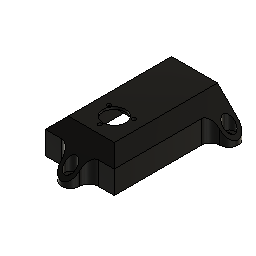
V205 Drybox Connector Buddy v2 (Autodesk Fusion 360 design; units mm, degrees)
Autodesk Fusion 360 part; units mm, degrees
sketch "Sketch7" plane through (0, 0, 0) normal (0, 0, 1) x (1, 0, 0)
  line L0 (30, -50) -> (-30, -50)
  line L1 (-30, -50) -> (-30, 50)
  line L2 (-30, 50) -> (30, 50)
  line L3 (30, 50) -> (30, -50)
  line L4 (30, -50) -> (-30, 50) construction
  line L5 (-30, -50) -> (30, 50) construction
  dimension "d21" = 60
  dimension "d22" = 100
  constraint horizontal L0
  constraint perpendicular L0 L1
  constraint parallel L0 L2
  constraint parallel L1 L3
  constraint coincident L4 origin
  constraint coincident L5 origin
  measures "d21" distance of L1.end L2.end
  measures "d22" distance of L0.end L1.end
extrude "Extrude13" add sketch "Sketch7" along normal blind 30 makes body 1
chamfer "Chamfer8" distance 10 angle 45 3 edges at (-30, 0, 30) (30, 0, 30) (0, -50, 30) tangent chain off on bodies 1
shell "Shell2" thickness 2 removed faces 1 at (-10, 16.6667, 0) on bodies 1
ref_plane "WorkPlane2" through (0, 0, 20) normal (0, 0, 1) x (1, 0, 0)
sketch "Sketch8" plane through (0, 0, 20) normal (0, 0, 1) x (1, 0, 0)
  line L0 (30, 50) -> (30, -50)
  line L1 (30, -50) -> (-30, -50)
  line L2 (-30, -50) -> (-30, 50)
  line L3 (-30, 50) -> (30, 50)
  line L4 (0, -50) -> (0, -58) construction
  circle A0 centre (0, -58) radius 8 construction
  circle A1 centre (38, 42) radius 8 construction
  circle A2 centre (-38, 42) radius 8 construction
  line L5 (30, 50) -> (38, 50)
  line L6 (-30, 50) -> (-38, 50)
  line L7 (38, 34) -> (30, 34)
  line L8 (-38, 34) -> (-30, 34)
  line L9 (8, -58) -> (8, -50)
  line L10 (-8, -58) -> (-8, -50)
  line L11 (8, -50) -> (-8, -50)
  line L12 (-8, -50) -> (-8, -66)
  line L13 (-8, -66) -> (8, -66)
  line L14 (8, -66) -> (8, -50)
  line L15 (8, -50) -> (-8, -66) construction
  line L16 (-8, -50) -> (8, -66) construction
  line L17 (30, 34) -> (46, 34)
  line L18 (46, 34) -> (46, 50)
  line L19 (46, 50) -> (30, 50)
  line L20 (30, 50) -> (30, 34)
  line L21 (30, 34) -> (46, 50) construction
  line L22 (46, 34) -> (30, 50) construction
  line L23 (-30, 34) -> (-46, 34)
  line L24 (-46, 34) -> (-46, 50)
  line L25 (-46, 50) -> (-30, 50)
  line L26 (-30, 50) -> (-30, 34)
  line L27 (-30, 34) -> (-46, 50) construction
  line L28 (-46, 34) -> (-30, 50) construction
  point P0 (0, -58)
  point P1 (38, 42)
  point P2 (-38, 42)
  dimension "d35" = 16
  constraint midpoint L1 L4.start
  constraint perpendicular L1 L4
  constraint coincident P0 L4.end
  constraint equal A1 A2
  constraint equal A0 A2
  constraint tangent L1 A0
  constraint tangent L0 A1
  constraint tangent L2 A2
  constraint coincident L0.start L3.end
  constraint perpendicular L0 L5
  constraint coincident L2.end L3.start
  constraint perpendicular L0 L6
  constraint coincident A2 L6.end
  constraint coincident A1 L5.end
  constraint tangent A1 L5
  constraint tangent A2 L6
  constraint coincident A1 L7.start
  constraint tangent A1 L7
  constraint coincident L0 L7.end
  constraint perpendicular L0 L7
  constraint coincident A2 L8.start
  constraint tangent A2 L8
  constraint coincident L2 L8.end
  constraint perpendicular L2 L8
  constraint coincident A0 L9.start
  constraint tangent A0 L9
  constraint coincident L1 L9.end
  constraint perpendicular L1 L9
  constraint coincident A0 L10.start
  constraint tangent A0 L10
  constraint coincident L1 L10.end
  constraint perpendicular L1 L10
  constraint horizontal L11
  constraint perpendicular L11 L12
  constraint parallel L11 L13
  constraint parallel L12 L14
  constraint coincident L15 P0
  constraint coincident L16 P0
  constraint horizontal L17
  constraint perpendicular L17 L18
  constraint parallel L17 L19
  constraint parallel L18 L20
  constraint coincident L21 P1
  constraint coincident L22 P1
  constraint coincident P1 A1.centre
  constraint horizontal L23
  constraint perpendicular L23 L24
  constraint parallel L23 L25
  constraint parallel L24 L26
  constraint coincident L27 P2
  constraint coincident L28 P2
  constraint coincident P2 A2.centre
  measures "d35" diameter of A0
extrude "Extrude14" add sketch "Sketch8" against normal up to surface (20 mm away) contours L0 L5 L7 L17 L18 L19 L20 | L2 L6 L8 L23 L24 L25 L26 | L1 L9 L10 L11 L12 L13 L14 bodies 1
chamfer "Chamfer9" distance 16 angle 45 3 edges at (-46, 42, 20) (46, 42, 20) (0, -66, 20) tangent chain off on bodies 1
sketch "Sketch9" plane through (0, 0, 30) normal (0, 0, 1) x (-1, 0, 0)
  line L0 (20, -50) -> (20, 40)
  line L1 (20, 40) -> (-20, 40)
  line L2 (-20, 40) -> (-20, -50)
  line L3 (-20, -50) -> (20, -50)
  line L4 (-8, 66) -> (-8, 50)
  line L5 (-30, 50) -> (-8, 50)
  line L6 (-30, -34) -> (-30, 50)
  line L7 (-30, -34) -> (-46, -34)
  line L8 (-46, -34) -> (-46, -50)
  line L9 (46, -50) -> (-46, -50)
  line L10 (46, -50) -> (46, -34)
  line L11 (46, -34) -> (30, -34)
  line L12 (30, 50) -> (30, -34)
  line L13 (8, 50) -> (30, 50)
  line L14 (8, 50) -> (8, 66)
  line L15 (8, 66) -> (-8, 66)
  line L16 (-38, -34) -> (-38, -50) construction
  line L17 (38, -34) -> (38, -50) construction
  line L18 (38, -42) -> (-38, -42) construction
  line L19 (-8, 58) -> (0, 58) construction
  line L20 (0, 58) -> (0, 66) construction
  constraint midpoint L7 L16.start
  constraint coincident L9 L16.end
  constraint perpendicular L9 L16
  constraint midpoint L11 L17.start
  constraint coincident L9 L17.end
  constraint perpendicular L9 L17
  constraint midpoint L17 L18.start
  constraint midpoint L16 L18.end
  constraint midpoint L4 L19.start
  constraint perpendicular L4 L19
  constraint perpendicular L15 L20
  constraint midpoint L15 L20.end
hole "Hole1" at (38, 42, 30) at (-38, 42, 30) at (0, -58, 30) direction (0, 0, -1) diameter 4.5 end through all counterbore diameter 10 counterbore depth 26 bodies 1
fillet "Fillet2" radius 8 6 edges at (8, -66, 2) (-8, -66, 2) (46, 34, 2) (46, 50, 2) (-46, 50, 2) (-46, 34, 2) on bodies 1
sketch "Sketch10" plane through (0, 0, 30) normal (0, 0, 1) x (-1, 0, 0)
  line L0 (20, -50) -> (20, 40)
  line L1 (20, 40) -> (-20, 40)
  line L2 (-20, 40) -> (-20, -50)
  line L3 (-20, -50) -> (20, -50)
  line L4 (0, 40) -> (0, 20) construction
  dimension "d46" = 20
  constraint midpoint L1 L4.start
  constraint perpendicular L1 L4
  measures "d46" distance of L4.start L4.end
hole "Hole2" at (0, -20, 30) direction (0, 0, -1) diameter 20 depth 30 tip angle 118 bodies 1
sketch "Sketch11" plane through (0, 0, 30) normal (0, 0, 1) x (-1, 0, 0)
  circle A0 centre (0, 20) radius 10
  line L0 (20, -50) -> (20, 40)
  line L1 (20, 40) -> (-20, 40)
  line L2 (-20, 40) -> (-20, -50)
  line L3 (-20, -50) -> (20, -50)
  line L4 (0, 20) -> (0, 32.5) construction
  point P0 (-10.8253, 13.75)
  point P1 (10.8253, 13.75)
  dimension "d54" = 12.5
  dimension "d56" = 360
  constraint coincident A0.centre L4.start
  constraint vertical L4
  measures "d54" distance of A0.centre L4.end
hole "Hole3" at (0, -32.5, 30) at (-10.8253, -13.75, 30) at (10.8253, -13.75, 30) direction (0, 0, -1) diameter 3.4 depth 30 tip angle 118 bodies 1
fillet "Fillet3" radius 8 4 edges at (-30, 34, 10) (-8, -50, 10) (8, -50, 10) (30, 34, 10) on bodies 1
sketch "Sketch12" plane through (0, 0, 4) normal (0, 0, 1) x (-1, 0, 0)
  circle A0 centre (0, 58) radius 5
  circle A1 centre (0, 58) radius 2.25
  circle A2 centre (-38, -42) radius 2.25
  circle A3 centre (38, -42) radius 2.25
  circle A4 centre (0, 58) radius 2.25
extrude "Extrude15" add sketch "Sketch12" against normal blind 0.3 contours A1 A4 | A2 | A3 bodies 1
ref_plane "WorkPlane3" through (0, 50, 15) normal (0, 1, 0) x (-1, 0, 0)
sketch "Sketch14" plane through (0, 50, 0) normal (0, 1, 0) x (1, 0, 0)
  line L0 (10, -5) -> (-10, -5)
  line L1 (-20, -15) -> (20, -15) construction
  arc A0 (-10, -5) -> (-14, -9) centre (-10, -9) ccw
  line L2 (14, -5) -> (-14, -25) construction
  line L3 (-14, -9) -> (-14, -20)
  line L4 (-9, -25) -> (9, -25)
  circle A1 centre (-20, -15) radius 1.75
  circle A2 centre (20, -15) radius 1.75
  line L5 (9, -25) -> (14, -20)
  line L6 (14, -25) -> (-14, -5) construction
  line L7 (0, 0) -> (0, -30) construction
  circle A3 centre (20, -15) radius 3.5 construction
  circle A4 centre (-20, -15) radius 3.5 construction
  line L8 (14, -20) -> (14, -9)
  arc A5 (14, -9) -> (10, -5) centre (10, -9) ccw
  line L9 (-14, -20) -> (-9, -25)
  line L10 (20, -30) -> (-20, -30)
  point P0 (0, -15)
  dimension "d66" = 20
  dimension "d67" = 28
  dimension "d68" = 3.5
  dimension "d69" = 40
  dimension "d70" = 5
  dimension "d71" = 5
  dimension "d72" = 4
  dimension "d73" = 4
  dimension "d74" = 7
  constraint coincident L7.start origin
  constraint perpendicular L0 L8
  constraint parallel L3 L8
  constraint parallel L0 L4
  constraint coincident P0 L6
  constraint coincident P0 L2
  constraint coincident P0 L7
  constraint perpendicular L1 L8
  constraint midpoint P0 L1
  constraint coincident L1.start A1.centre
  constraint coincident L1.end A2.centre
  constraint equal A1 A2
  constraint coincident L2.end L3
  constraint coincident L2.end L4
  constraint coincident L6.start L4
  constraint coincident L6.start L8
  constraint perpendicular L5 L9
  constraint equal L5 L9
  constraint coincident L6.end L3
  constraint coincident L6.end L0
  constraint tangent A0 L3
  constraint tangent L0 A0
  constraint coincident L2.start L0
  constraint coincident L2.start L8
  constraint tangent L0 A5
  constraint tangent L8 A5
  constraint concentric A1 A4
  constraint concentric A2 A3
  constraint equal A3 A4
  constraint vertical L7
  constraint midpoint P0 L7
  constraint horizontal L0
  constraint midpoint L7.end L10
  measures "d66" distance of L6.end L2.end
  measures "d67" distance of L6.start L2.end
  measures "d68" diameter of A1
  measures "d69" distance of L1.start L1.end
  measures "d70" distance of L3.end L2.end
  measures "d71" distance of L4.start L2.end
  measures "d72" radius of A0
  measures "d73" radius of A5
  measures "d74" diameter of A4
extrude "Extrude16" cut sketch "Sketch14" against normal blind 2 bodies 1
ref_plane "WorkPlane4" through (0, -3, 9.5858) normal (0, 1, 0) x (-1, 0, 0)
sketch "Sketch15" plane through (0, -3, 0) normal (0, 1, 0) x (1, 0, 0)
  line L0 (-30, -20) -> (-20, -30)
  line L1 (-20, -30) -> (20, -30)
  line L2 (20, -30) -> (30, -20)
  line L3 (30, -20) -> (30, 0)
  line L4 (30, 0) -> (28, 0)
  line L5 (28, 0) -> (28, -19.1716)
  line L6 (28, -19.1716) -> (19.1716, -28)
  line L7 (19.1716, -28) -> (-19.1716, -28)
  line L8 (-19.1716, -28) -> (-28, -19.1716)
  line L9 (-28, -19.1716) -> (-28, 0)
  line L10 (-28, 0) -> (-30, 0)
  line L11 (-30, 0) -> (-30, -20)
  line L12 (28, -19.1716) -> (-28, -19.1716)
  constraint coincident L5.end L6.start
  constraint coincident L8.end L9.start
extrude "Extrude17" add sketch "Sketch15" along normal blind 2 contours L6 L7 L8 L12 bodies 1
ref_plane "WorkPlane1" through (0, 50, 15) normal (0, 1, 0) x (-1, 0, 0) in component "support"
sketch "Sketch1" plane through (0, 50, 0) normal (0, 1, 0) x (1, 0, 0) in component "support"
  arc A0 (14, -9) -> (10, -5) centre (10, -9) ccw
  arc A1 (-10, -5) -> (-14, -9) centre (-10, -9) ccw
  line L0 (-10, -5) -> (10, -5)
  line L1 (9, -25) -> (-9, -25)
  line L2 (14, -20) -> (9, -25)
  circle A2 centre (20, -15) radius 1.75
  line L3 (9, -25) -> (-9, -25)
  line L4 (-9, -25) -> (-14, -20)
  line L5 (-14, -20) -> (-14, -9)
  arc A3 (-10, -5) -> (-14, -9) centre (-10, -9) ccw
  line L6 (-10, -5) -> (10, -5)
  arc A4 (14, -9) -> (10, -5) centre (10, -9) ccw
  line L7 (14, -9) -> (14, -20)
  line L8 (14, -20) -> (9, -25)
  circle A5 centre (-20, -15) radius 1.75
  line L9 (-38, 0) -> (-38, -12)
  line L10 (-38, -12) -> (-20, -30)
  line L11 (-20, -30) -> (20, -30)
  line L12 (20, -30) -> (38, -12)
  line L13 (38, -12) -> (38, 0)
  line L14 (38, 0) -> (-38, 0)
  line L15 (-13.75, -19.8964) -> (-13.75, -9)
  arc A6 (-10, -5.25) -> (-13.75, -9) centre (-10, -9) ccw
  line L16 (-10, -5.25) -> (10, -5.25)
  arc A7 (13.75, -9) -> (10, -5.25) centre (10, -9) ccw
  line L17 (13.75, -9) -> (13.75, -19.8964)
  line L18 (13.75, -19.8964) -> (8.8964, -24.75)
  line L19 (8.8964, -24.75) -> (-8.8964, -24.75)
  line L20 (-8.8964, -24.75) -> (-13.75, -19.8964)
  line L21 (0, -44.5) -> (0, -5)
  line L22 (-10, -5.25) -> (-5, -24.75)
  line L23 (10, -5.25) -> (5, -24.75)
  point P0 (0, -24.75)
  dimension "d84" = 0.25
  dimension "d87" = 10
  constraint midpoint L21 P0
  constraint coincident L19 P0
  constraint coincident L6 L21.end
  constraint perpendicular L6 L21
  constraint symmetric L21 L22 L23
  constraint coincident L19 L23.end
  constraint coincident L19 L22.end
  constraint coincident A6.start L16.start
  constraint coincident L16.end A7.end
  measures "d87" distance of L22.end L23.end
extrude "Extrude1" add sketch "Sketch1" against normal blind 2 separate body contours L16 L19 L21 L22 | L16 L19 L21 L23 makes body 2 in component "support"
component "support" placed x (1, 0, 0) y (0, 1, 0) z (0, 0, 1) at (0, 0, 0)
